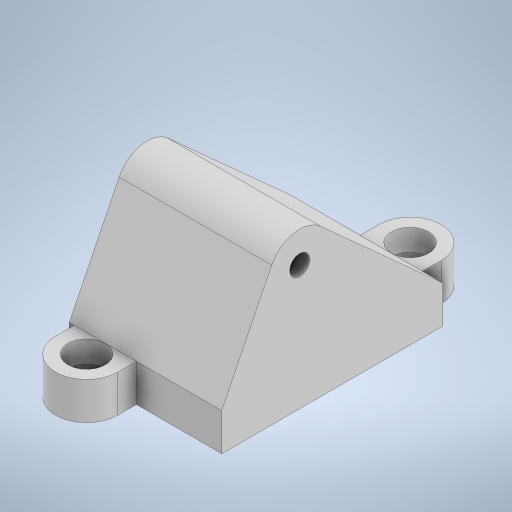
# Autodesk Inventor part: uchwyt_gorny
Saved by Autodesk Inventor 2023 (Build 270158000, 158)
## iProperties
Created: 2024-05-12
Part Number: uchwyt_gorny
Material: Ogólny
Document SubType Name: Modeling
Designer: kamil
Density: 1 g/cm^3
Appearance: Domyślna
Author: kamil
Autodesk Inventor part; units mm, degrees
ref_plane "YZ Plane" through (0, 0, 0) normal (1, 0, 0) x (0, 1, 0)
ref_plane "XZ Plane" through (0, 0, 0) normal (0, 1, 0) x (-1, 0, 0)
ref_plane "XY Plane" through (0, 0, 0) normal (0, 0, 1) x (1, 0, 0)
sketch "Szkic1" plane through (0, 0, 0) normal (0, 1, 0) x (-1, 0, 0)
  circle A0 centre (-11.25, -20.75) radius 3
  circle A1 centre (-0.8, 20.75) radius 3
  line L0 (5, -17.75) -> (-6.25, -17.75)
  line L1 (5, -17.75) -> (5, 17.75)
  line L2 (5, 17.75) -> (4.2, 17.75)
  line L3 (4.2, 20.75) -> (4.2, 17.75)
  arc A2 (4.2, 20.75) -> (-5.8, 20.75) centre (-0.8, 20.75) ccw
  line L4 (-5.8, 17.75) -> (-5.8, 20.75)
  line L5 (-5.8, 17.75) -> (-19.5, 17.75)
  line L6 (-19.5, -17.75) -> (-19.5, 17.75)
  line L7 (-16.25, -17.75) -> (-19.5, -17.75)
  line L8 (-16.25, -20.75) -> (-16.25, -17.75)
  arc A3 (-16.25, -20.75) -> (-6.25, -20.75) centre (-11.25, -20.75) ccw
  line L9 (-6.25, -17.75) -> (-6.25, -20.75)
  point P0 (0, 0)
  point P1 (0, 0)
  constraints: 20 end point, 4 centre point, 4 point on circle
extrude "Wyciągnięcie proste1" add sketch "Szkic1" along normal blind 6
sketch "Szkic2" plane through (0, 0, 0) normal (0, -1, 0) x (1, 0, 0)
  circle A0 centre (0.8, 20.75) radius 3 projected
  circle A1 centre (11.25, -20.75) radius 3 projected
  circle A2 centre (11.25, -20.75) radius 1.6
  circle A3 centre (0.8, 20.75) radius 1.6
  point P0 (0, 0)
  dimension "d3" = 3.2
  dimension "d4" = 3.2
  constraints: 2 centre point, 2 coincident
  measures "d3" diameter of A2
  measures "d4" diameter of A3
extrude "Wyciągnięcie proste2" add sketch "Szkic2" against normal blind 2.5
sketch "Szkic3" plane through (-5, 0, -17.75) normal (-1, 0, 0) x (0, 0, 1)
  line L0 (0, 0) -> (0, 6) projected
  line L1 (35.5, 0) -> (35.5, 6) projected
  line L2 (35.5, 0) -> (0, 0) construction
  line L3 (23, 0) -> (23, 20) construction
  circle A0 centre (23, 20) radius 5
  line L4 (0, 6) -> (19.6524, 23.714)
  line L5 (35.5, 6) -> (27.4821, 22.2161)
  line L6 (0, 6) -> (35.5, 6) projected
  point P0 (17.75, 0)
  dimension "d7" = 12.5
  dimension "d8" = 20
  dimension "d9" = 10
  constraints: 6 end point, 2 coincident, 2 point on circle, 2 tangent, 1 centre point, 1 point on line, 1 vertical
  measures "d7" distance between parallel lines of L1 L3
  measures "d8" distance of L3.start L3.end
  measures "d9" diameter of A0
extrude "Wyciągnięcie proste3" add sketch "Szkic3" against normal up to surface (24.5 mm away)
sketch "Szkic4" plane through (-5, 0, -17.75) normal (-1, 0, 0) x (0, 0, 1)
  line L0 (0, 0) -> (35.5, 0) projected
  line L1 (35.5, 0) -> (35.5, 6) projected
  line L2 (35.5, 6) -> (27.4821, 22.2161) projected
  arc A0 (27.4821, 22.2161) -> (19.6524, 23.714) centre (23, 20) ccw projected
  line L3 (19.6524, 23.714) -> (0, 6) projected
  line L4 (0, 0) -> (0, 6) projected
  point P0 (17.75, 0)
hole "Otwór1" at (-5, 20, 5.25) direction (1, 0, 0) diameter 3.2 end through all
